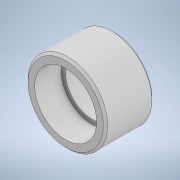
# Autodesk Inventor part: MotorBeltTensionerRoller 10mm
Saved by Autodesk Inventor 2022.2 (Build 262287000, 287)
## iProperties
Created: 2022-01-06
Part Number: MotorBeltTensionerRoller 10mm
Material: Generic
Document SubType Name: Modeling
Designer: Jochen
Density: 1 g/cm^3
Appearance: Default
Author: Jochen
Autodesk Inventor part; units mm, degrees
ref_plane "YZ Plane" through (0, 0, 0) normal (1, 0, 0) x (0, 1, 0)
ref_plane "XZ Plane" through (0, 0, 0) normal (0, 1, 0) x (-1, 0, 0)
ref_plane "XY Plane" through (0, 0, 0) normal (0, 0, 1) x (1, 0, 0)
sketch "Sketch1" plane through (0, 0, 0) normal (0, 0, 1) x (1, 0, 0)
  line L0 (-6.3, 0) -> (6.3, 0) construction
  line L1 (0, -6.3) -> (0, 6.3) construction
  circle A0 centre (0, 0) radius 3.5
  circle A1 centre (0, 0) radius 4.5
  circle A2 centre (0, 0) radius 3
  dimension "d0" = 7
  dimension "d1" = 9
  dimension "d6" = 6
  constraints: 3 centre point, 3 coincident
  measures "d0" diameter of A0
  measures "d1" diameter of A1
  measures "d6" diameter of A2
extrude "Extrusion1" add sketch "Sketch1" along normal blind 2.5 contours A0 | A1
extrude "Extrusion2" add sketch "Sketch1" along normal blind 3 from surface at 2.5 contours A1
chamfer "Chamfer1" distance 0.25 angle 45 2 edges at (-4.5, 0, 0) (-4.5, 0, 5.5)
body "Solid1"
